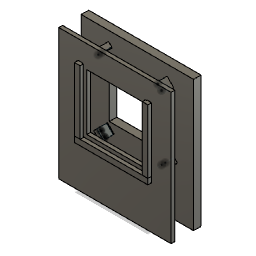
Target holder complete v23 (Autodesk Fusion 360 design; units mm, degrees)
Autodesk Fusion 360 part; units mm, degrees
sketch "Sketch1" plane through (0, 0, 0) normal (0, 0, 1) x (1, 0, 0) in component "Faceplate"
  line L0 (10, 10) -> (310, 10)
  line L1 (310, 10) -> (310, 360)
  line L2 (310, 360) -> (10, 360)
  line L3 (10, 360) -> (10, 10)
  line L4 (85, 300) -> (235, 300)
  line L5 (235, 300) -> (235, 150)
  line L6 (235, 150) -> (85, 150)
  line L7 (85, 150) -> (85, 300)
  dimension "d7" = 10
  dimension "d8" = 10
  dimension "d10" = 350
  dimension "d11" = 75
  dimension "d12" = 140
  dimension "d13" = 150
  dimension "d14" = 150
  dimension "d15" = 75
  constraint horizontal L0
  constraint vertical L1
  constraint horizontal L2
  constraint vertical L3
  constraint horizontal L4
  constraint vertical L5
  constraint horizontal L6
  constraint vertical L7
  measures "d7" horizontal distance of origin L0.start
  measures "d8" vertical distance of origin L0.start
  measures "d10" distance of L0.end L1.end
  measures "d11" horizontal distance of L0.start L6.end
  measures "d12" vertical distance of L0.start L6.end
  measures "d13" distance of L5.end L6.end
  measures "d14" distance of L4.end L5.end
  measures "d15" horizontal distance of L0.end L5.end
extrude "Extrude1" add sketch "Sketch1" against normal blind 10 makes body 1 in component "Faceplate"
sketch "Sketch2" plane through (0, 0, 0) normal (0, 0, 1) x (1, 0, 0) in component "Bottom holder"
  line L0 (235, 150) -> (85, 150)
  line L1 (85, 150) -> (85, 300)
  line L2 (85, 300) -> (235, 300)
  line L3 (235, 300) -> (235, 150)
  line L4 (10, 360) -> (10, 10)
  line L5 (10, 10) -> (310, 10)
  line L6 (310, 10) -> (310, 360)
  line L7 (310, 360) -> (10, 360)
  line L8 (258, 125) -> (62, 125)
  line L9 (62, 125) -> (62, 140)
  line L10 (62, 140) -> (258, 140)
  line L11 (258, 125) -> (258, 140)
  dimension "d18" = 196
  dimension "d20" = 15
  dimension "d69" = 10
  dimension "d70" = 23
  dimension "d74" = 15
  constraint horizontal L8
  constraint vertical L9
  constraint perpendicular L9 L10
  constraint perpendicular L10 L11
  measures "d18" distance of L8.start L8.end
  measures "d20" distance of L9.end L8.end
  measures "d69" vertical distance of L0.start L10.end
  measures "d70" horizontal distance of L0.end L9.end
  measures "d74" distance of L8.start L10.end
sketch "Sketch1 (2)" plane through (0, 0, 0) normal (0, 0, 1) x (1, 0, 0) in component "Left holder"
  line L0 (235, 150) -> (85, 150)
  line L1 (85, 150) -> (85, 300)
  line L2 (85, 300) -> (235, 300)
  line L3 (235, 300) -> (235, 150)
  line L4 (10, 360) -> (10, 10)
  line L5 (10, 10) -> (310, 10)
  line L6 (310, 10) -> (310, 360)
  line L7 (310, 360) -> (10, 360)
  line L8 (77, 310) -> (62, 310)
  line L9 (62, 310) -> (62, 140)
  line L10 (62, 140) -> (77, 140)
  line L11 (77, 140) -> (77, 310)
  dimension "d23" = 15
  dimension "d24" = 170
  dimension "d64" = 10
  dimension "d72" = 8
  constraint horizontal L8
  constraint vertical L9
  constraint horizontal L10
  constraint vertical L11
  measures "d23" distance of L8.start L8.end
  measures "d24" distance of L8.end L9.end
  measures "d64" vertical distance of L0.end L10.end
  measures "d72" horizontal distance of L1.end L8.start
sketch "Sketch1 (3)" plane through (0, 0, 0) normal (0, 0, 1) x (1, 0, 0) in component "Right holder"
  line L0 (235, 150) -> (85, 150)
  line L1 (85, 150) -> (85, 300)
  line L2 (85, 300) -> (241.0837, 300)
  line L3 (235, 300) -> (235, 150)
  line L4 (10, 360) -> (10, 10)
  line L5 (10, 10) -> (310, 10)
  line L6 (310, 10) -> (310, 360)
  line L7 (310, 360) -> (10, 360)
  line L8 (258, 310) -> (258, 140)
  line L9 (243, 140) -> (243, 310)
  line L10 (243, 140) -> (258, 140)
  line L11 (258, 310) -> (243, 310)
  dimension "d21" = 15
  dimension "d66" = 10
  dimension "d67" = 170
  dimension "d73" = 8
  constraint vertical L8
  constraint vertical L9
  constraint perpendicular L8 L10
  constraint perpendicular L9 L11
  measures "d21" distance of L9.end L8.start
  measures "d66" vertical distance of L0.start L9.start
  measures "d67" distance of L8.start L8.end
  measures "d73" horizontal distance of L3.start L9.end
extrude "Extrude2" add sketch "Sketch2" along normal blind 10 separate body contours L8 L9 L10 L11 makes body 2 in component "Bottom holder"
extrude "Extrude1'" add sketch "Sketch1 (2)" along normal blind 10 separate body contours L8 L9 L10 L11 makes body 3 in component "Left holder"
extrude "Extrude1''" add sketch "Sketch1 (3)" along normal blind 10 separate body contours L8 L9 L10 L11 makes body 4 in component "Right holder"
sketch "Sketch2 (2)" plane through (77, 0, 0) normal (1, 0, 0) x (0, 0, -1) in component "Left holder"
  line L0 (0, 140) -> (0, 310)
  line L1 (0, 310) -> (-10, 310)
  line L2 (-10, 310) -> (-10, 140)
  line L3 (-10, 140) -> (0, 140)
  line L4 (0, 310) -> (-1.5, 310)
  line L5 (-1.5, 310) -> (-1.5, 140)
  line L6 (-1.5, 140) -> (0, 140)
  line L7 (0, 140) -> (0, 310)
  dimension "d31" = 1.5
  constraint horizontal L4
  constraint vertical L5
  constraint horizontal L6
  constraint vertical L7
  constraint coincident L3 L5.end
  constraint coincident L0.end L1.start
  measures "d31" distance of L0.end L4.end
extrude "Extrude2'" cut sketch "Sketch2 (2)" against normal blind 3 contours L0 L1 L3 L4 L5 L6 L7 bodies 3 in component "Left holder"
sketch "Sketch2 (3)" plane through (243, 0, 0) normal (-1, 0, 0) x (0, 0, 1) in component "Right holder"
  line L0 (0, 310) -> (0, 140)
  line L1 (10, 140) -> (10, 310)
  line L2 (0, 310) -> (1.5, 310)
  line L3 (1.5, 310) -> (1.5, 145)
  line L4 (1.5, 145) -> (0, 145)
  line L5 (0, 145) -> (0, 310)
  line L6 (0, 140) -> (10, 140)
  line L7 (10, 310) -> (0, 310)
  dimension "d34" = 1.5
  constraint horizontal L2
  constraint vertical L3
  constraint horizontal L4
  constraint vertical L5
  constraint coincident L0.start L2.start
  measures "d34" distance of L3.end L4.end
extrude "Extrude2''" cut sketch "Sketch2 (3)" against normal blind 3 contours L0 L2 L3 L4 L5 L7 bodies 4 in component "Right holder"
sketch "Sketch3" plane through (0, 0, 0) normal (0, 0, -1) x (-1, 0, 0) in component "Bottom holder"
  line L0 (-258, 125) -> (-62, 125)
  line L1 (-62, 125) -> (-62, 140)
  circle A0 centre (-218, 132.5) radius 2.25
  circle A1 centre (-102, 132.5) radius 2.25
  line L2 (-62, 140) -> (-258, 140)
  line L3 (-258, 140) -> (-258, 125)
  dimension "d37" = 40
  dimension "d38" = 7.5
  dimension "d39" = 40
  dimension "d40" = 7.5
  dimension "d41" = 4.5
  dimension "d42" = 4.5
  measures "d37" horizontal distance of L0.start A0.centre
  measures "d38" vertical distance of L0.start A0.centre
  measures "d39" horizontal distance of L0.end A1.centre
  measures "d40" vertical distance of L0.end A1.centre
  measures "d41" diameter of A1
  measures "d42" diameter of A0
extrude "Extrude3" cut sketch "Sketch3" against normal blind 7 contours A0 | A1 bodies 2 in component "Bottom holder"
sketch "Sketch3 (2)" plane through (0, 0, 0) normal (0, 0, -1) x (-1, 0, 0) in component "Left holder"
  line L0 (-74, 310) -> (-74, 140)
  line L1 (-74, 140) -> (-62, 140)
  line L2 (-62, 140) -> (-62, 310)
  line L3 (-62, 310) -> (-74, 310)
  circle A0 centre (-68.5, 290) radius 2.25
  circle A1 centre (-68.5, 160) radius 2.25
  dimension "d45" = 20
  dimension "d46" = 20
  dimension "d47" = 6.5
  dimension "d48" = 6.5
  dimension "d49" = 4.5
  dimension "d50" = 4.5
  measures "d45" vertical distance of L2.end A0.centre
  measures "d46" vertical distance of L1.end A1.centre
  measures "d47" horizontal distance of L2.end A0.centre
  measures "d48" horizontal distance of L1.end A1.centre
  measures "d49" diameter of A0
  measures "d50" diameter of A1
sketch "Sketch3 (3)" plane through (0, 0, 0) normal (0, 0, -1) x (-1, 0, 0) in component "Right holder"
  line L0 (-246, 145) -> (-246, 310)
  line L1 (-258, 310) -> (-258, 140)
  circle A0 centre (-251.5, 290) radius 2.25
  circle A1 centre (-251.5, 160) radius 2.25
  line L2 (-246, 310) -> (-258, 310)
  line L3 (-258, 140) -> (-243, 140)
  line L4 (-243, 140) -> (-243, 145)
  line L5 (-243, 145) -> (-246, 145)
  dimension "d52" = 20
  dimension "d53" = 20
  dimension "d55" = 6.5
  dimension "d56" = 6.5
  dimension "d57" = 4.5
  dimension "d58" = 4.5
  measures "d52" vertical distance of L1.start A0.centre
  measures "d53" vertical distance of L1.end A1.centre
  measures "d55" horizontal distance of L1.start A0.centre
  measures "d56" horizontal distance of L1.end A1.centre
  measures "d57" diameter of A1
  measures "d58" diameter of A0
extrude "Extrude3'" cut sketch "Sketch3 (2)" against normal blind 7 contours A0 | A1 bodies 3 in component "Left holder"
extrude "Extrude3''" cut sketch "Sketch3 (3)" against normal blind 7 contours A0 | A1 bodies 4 in component "Right holder"
ref_plane "WorkPlane1" through (160, 185, -60) normal (0, 0, -1) x (-1, 0, 0) in component "Bottom holder"
sketch "Sketch1 (4)" plane through (160, 185, -60) normal (0, 0, -1) x (1, 0, 0) in component "Backplate"
  line L0 (150, -175) -> (-150, -175)
  line L1 (-150, -175) -> (-150, 175)
  line L2 (-150, 175) -> (150, 175)
  line L3 (150, 175) -> (150, -175)
  line L4 (75, -115) -> (-75, -115)
  line L5 (-75, -115) -> (-75, 35)
  line L6 (-75, 35) -> (75, 35)
  line L7 (75, 35) -> (75, -115)
  dimension "d76" = 300
  dimension "d77" = 350
  dimension "d78" = 175
  dimension "d79" = 150
  dimension "d84" = 150
  dimension "d85" = 150
  dimension "d86" = 75
  dimension "d87" = 60
  constraint horizontal L0
  constraint vertical L1
  constraint horizontal L2
  constraint vertical L3
  constraint horizontal L4
  constraint vertical L5
  constraint horizontal L6
  constraint vertical L7
  measures "d76" distance of L1.end L2.end
  measures "d77" distance of L0.start L2.end
  measures "d78" vertical distance of origin L1.end
  measures "d79" horizontal distance of origin L1.end
  measures "d84" distance of L4.start L6.end
  measures "d85" distance of L4.start L4.end
  measures "d86" distance of L3 L6.end
  measures "d87" distance of L0 L4.start
extrude "Extrude1'''" add sketch "Sketch1 (4)" along normal blind 20 separate body makes body 5 in component "Backplate"
sketch "Sketch1 (5)" plane through (0, 0, -60) normal (0, 0, 1) x (1, 0, 0) in component "Help lines"
  line L0 (235, 150) -> (85, 150)
  line L1 (85, 150) -> (85, 300)
  line L2 (85, 300) -> (235, 300)
  line L3 (235, 300) -> (235, 150)
  line L4 (10, 10) -> (310, 10)
  line L5 (310, 10) -> (310, 360)
  line L6 (310, 360) -> (10, 360)
  line L7 (10, 360) -> (10, 10)
  line L8 (85, 300) -> (235, 150)
  line L9 (85, 150) -> (235, 300)
  circle A0 centre (160, 225) radius 115
  dimension "d90" = 230
  constraint coincident L1.end L2.start
  constraint coincident L0.start L3.end
  constraint coincident L0.end L1.start
  constraint coincident L2.end L3.start
  constraint midpoint L8 A0.centre
  measures "d90" diameter of A0
sketch "Sketch2 (4)" plane through (0, 0, -60) normal (0, 0, 1) x (1, 0, 0) in component "Sensor-Holder West"
  line L0 (235, 150) -> (85, 150)
  line L1 (85, 150) -> (85, 300)
  line L2 (85, 300) -> (235, 300)
  line L3 (235, 300) -> (235, 150)
  line L4 (10, 10) -> (310, 10)
  line L5 (310, 10) -> (310, 360)
  line L6 (310, 360) -> (10, 360)
  line L7 (10, 360) -> (10, 10)
  line L8 (78.8806, 143.4853) -> (96.5583, 125.8076)
  line L9 (96.5583, 125.8076) -> (88.073, 117.3223)
  line L10 (88.073, 117.3223) -> (70.3954, 135)
  line L11 (70.3954, 135) -> (78.8806, 143.4853)
  circle A0 centre (160, 225) radius 115
  point P0 (85, 150)
  dimension "d91" = 12
  dimension "d92" = 25
  dimension "d93" = 15
  dimension "d94" = 45
  constraint perpendicular L8 L9
  constraint parallel L8 L10
  constraint parallel L9 L11
  constraint coincident L8.start A0
  measures "d91" distance of L8.start L10.end
  measures "d92" distance of L9.end L10.end
  measures "d93" vertical distance of L10.end P0
  measures "d94" angle of L7 L10
extrude "Extrude1''''" add sketch "Sketch2 (4)" along normal blind 27 separate body contours L8 L9 L10 L11 makes body 6 in component "Sensor-Holder West"
sketch "Sketch3 (4)" plane through (111.183, 111.183, 0) normal (0.707107, 0.707107, 0) x (0, 0, -1) in component "Sensor-Holder West"
  line L0 (60, 20.6824) -> (60, 45.6824)
  line L1 (60, 45.6824) -> (33, 45.6824)
  line L2 (33, 45.6824) -> (33, 20.6824)
  line L3 (33, 20.6824) -> (60, 20.6824)
  line L4 (60, 45.6824) -> (59, 45.6824)
  line L5 (59, 45.6824) -> (59, 20.6824)
  line L6 (59, 20.6824) -> (60, 20.6824)
  line L7 (60, 20.6824) -> (60, 45.6824)
  point P0 (60, 45.9619)
  dimension "d97" = 1
  constraint horizontal L4
  constraint vertical L5
  constraint horizontal L6
  constraint vertical L7
  constraint coincident L3 L5.end
  constraint coincident L0.end L1.start
  measures "d97" horizontal distance of L4.end P0
extrude "Extrude2'''" add sketch "Sketch3 (4)" along normal blind 2 contours L0 L1 L3 L4 L5 L6 L7 bodies 6 in component "Sensor-Holder West"
sketch "Sketch4" plane through (111.183, 111.183, 0) normal (0.707107, 0.707107, 0) x (0, 0, -1) in component "Sensor-Holder West"
  line L0 (59, 20.6824) -> (59, 45.6824)
  line L1 (59, 45.6824) -> (33, 45.6824)
  line L2 (33, 45.6824) -> (33, 20.6824)
  line L3 (33, 20.6824) -> (59, 20.6824)
  circle A0 centre (38.5, 38.6824) radius 1.5
  circle A1 centre (38.5, 24.6824) radius 1.5
  dimension "d100" = 3
  dimension "d101" = 3
  dimension "d102" = 14
  dimension "d103" = 20.5
  dimension "d104" = 7
  dimension "d105" = 20.5
  measures "d100" diameter of A0
  measures "d101" diameter of A1
  measures "d102" distance of A0.centre A1.centre
  measures "d103" horizontal distance of L0.end A0.centre
  measures "d104" vertical distance of L1.end A0.centre
  measures "d105" horizontal distance of L0.start A1.centre
extrude "Extrude3'''" add sketch "Sketch4" along normal blind 3 contours A0 bodies 6 in component "Sensor-Holder West"
extrude "Extrude4" add sketch "Sketch4" along normal up to surface (3 mm away) contours A1 bodies 6 in component "Sensor-Holder West"
sketch "Sketch2 (5)" plane through (0, 0, -60) normal (0, 0, 1) x (1, 0, 0) in component "Sensor-Holder East"
  line L0 (235, 150) -> (85, 150)
  line L1 (85, 150) -> (85, 300)
  line L2 (85, 300) -> (235, 300)
  line L3 (235, 300) -> (235, 150)
  line L4 (10, 10) -> (310, 10)
  line L5 (310, 10) -> (310, 360)
  line L6 (310, 360) -> (10, 360)
  line L7 (10, 360) -> (10, 10)
  line L8 (78.8806, 143.4853) -> (96.5583, 125.8076)
  line L9 (96.5583, 125.8076) -> (88.073, 117.3223)
  line L10 (88.073, 117.3223) -> (70.3954, 135)
  line L11 (70.3954, 135) -> (78.8806, 143.4853)
  circle A0 centre (160, 225) radius 115
  point P0 (85, 150)
  dimension "d91_1" = 12
  dimension "d92_1" = 25
  dimension "d93_1" = 15
  dimension "d94_1" = 45
  constraint perpendicular L8 L9
  constraint parallel L8 L10
  constraint parallel L9 L11
  constraint coincident L8.start A0
  measures "d91_1" distance of L8.start L10.end
  measures "d92_1" distance of L9.end L10.end
  measures "d93_1" vertical distance of L10.end P0
  measures "d94_1" angle of L7 L10
extrude "Extrude1'''''" add sketch "Sketch2 (5)" along normal blind 27 separate body contours L8 L9 L10 L11 makes body 7 in component "Sensor-Holder East"
sketch "Sketch3 (5)" plane through (111.183, 111.183, 0) normal (0.707107, 0.707107, 0) x (0, 0, -1) in component "Sensor-Holder East"
  line L0 (60, 20.6824) -> (60, 45.6824)
  line L1 (60, 45.6824) -> (33, 45.6824)
  line L2 (33, 45.6824) -> (33, 20.6824)
  line L3 (33, 20.6824) -> (60, 20.6824)
  line L4 (60, 45.6824) -> (59, 45.6824)
  line L5 (59, 45.6824) -> (59, 20.6824)
  line L6 (59, 20.6824) -> (60, 20.6824)
  line L7 (60, 20.6824) -> (60, 45.6824)
  point P0 (60, 45.9619)
  dimension "d97_1" = 1
  constraint horizontal L4
  constraint vertical L5
  constraint horizontal L6
  constraint vertical L7
  constraint coincident L3 L5.end
  constraint coincident L0.end L1.start
  measures "d97_1" horizontal distance of L4.end P0
extrude "Extrude2''''" add sketch "Sketch3 (5)" along normal blind 2 contours L0 L1 L3 L4 L5 L6 L7 bodies 7 in component "Sensor-Holder East"
sketch "Sketch4 (2)" plane through (111.183, 111.183, 0) normal (0.707107, 0.707107, 0) x (0, 0, -1) in component "Sensor-Holder East"
  line L0 (59, 20.6824) -> (59, 45.6824)
  line L1 (59, 45.6824) -> (33, 45.6824)
  line L2 (33, 45.6824) -> (33, 20.6824)
  line L3 (33, 20.6824) -> (59, 20.6824)
  circle A0 centre (38.5, 38.6824) radius 1.5
  circle A1 centre (38.5, 24.6824) radius 1.5
  dimension "d100_1" = 3
  dimension "d101_1" = 3
  dimension "d102_1" = 14
  dimension "d103_1" = 20.5
  dimension "d104_1" = 7
  dimension "d105_1" = 20.5
  measures "d100_1" diameter of A0
  measures "d101_1" diameter of A1
  measures "d102_1" distance of A0.centre A1.centre
  measures "d103_1" horizontal distance of L0.end A0.centre
  measures "d104_1" vertical distance of L1.end A0.centre
  measures "d105_1" horizontal distance of L0.start A1.centre
extrude "Extrude3''''" add sketch "Sketch4 (2)" along normal blind 3 contours A0 bodies 7 in component "Sensor-Holder East"
extrude "Extrude4'" add sketch "Sketch4 (2)" along normal up to surface (3 mm away) contours A1 bodies 7 in component "Sensor-Holder East"
move_body "Move1" bodies 7 to x (1, 0, 0) y (0, 1, 0) z (0, 0, 1) at (2.1213, 2.1213, 0) in component "Sensor-Holder East"
sketch "Sketch2 (6)" plane through (0, 0, -60) normal (0, 0, 1) x (1, 0, 0) in component "Sensor-Holder South"
  line L0 (235, 150) -> (85, 150)
  line L1 (85, 150) -> (85, 300)
  line L2 (85, 300) -> (235, 300)
  line L3 (235, 300) -> (235, 150)
  line L4 (10, 10) -> (310, 10)
  line L5 (310, 10) -> (310, 360)
  line L6 (310, 360) -> (10, 360)
  line L7 (10, 360) -> (10, 10)
  line L8 (78.8806, 143.4853) -> (96.5583, 125.8076)
  line L9 (96.5583, 125.8076) -> (88.073, 117.3223)
  line L10 (88.073, 117.3223) -> (70.3954, 135)
  line L11 (70.3954, 135) -> (78.8806, 143.4853)
  circle A0 centre (160, 225) radius 115
  point P0 (85, 150)
  dimension "d91_2" = 12
  dimension "d92_2" = 25
  dimension "d93_2" = 15
  dimension "d94_2" = 45
  constraint perpendicular L8 L9
  constraint parallel L8 L10
  constraint parallel L9 L11
  constraint coincident L8.start A0
  measures "d91_2" distance of L8.start L10.end
  measures "d92_2" distance of L9.end L10.end
  measures "d93_2" vertical distance of L10.end P0
  measures "d94_2" angle of L7 L10
extrude "Extrude1''''''" add sketch "Sketch2 (6)" along normal blind 27 separate body contours L8 L9 L10 L11 makes body 8 in component "Sensor-Holder South"
sketch "Sketch3 (6)" plane through (111.183, 111.183, 0) normal (0.707107, 0.707107, 0) x (0, 0, -1) in component "Sensor-Holder South"
  line L0 (60, 20.6824) -> (60, 45.6824)
  line L1 (60, 45.6824) -> (33, 45.6824)
  line L2 (33, 45.6824) -> (33, 20.6824)
  line L3 (33, 20.6824) -> (60, 20.6824)
  line L4 (60, 45.6824) -> (59, 45.6824)
  line L5 (59, 45.6824) -> (59, 20.6824)
  line L6 (59, 20.6824) -> (60, 20.6824)
  line L7 (60, 20.6824) -> (60, 45.6824)
  point P0 (60, 45.9619)
  dimension "d97_2" = 1
  constraint horizontal L4
  constraint vertical L5
  constraint horizontal L6
  constraint vertical L7
  constraint coincident L3 L5.end
  constraint coincident L0.end L1.start
  measures "d97_2" horizontal distance of L4.end P0
extrude "Extrude2'''''" add sketch "Sketch3 (6)" along normal blind 2 contours L0 L1 L3 L4 L5 L6 L7 bodies 8 in component "Sensor-Holder South"
sketch "Sketch4 (3)" plane through (111.183, 111.183, 0) normal (0.707107, 0.707107, 0) x (0, 0, -1) in component "Sensor-Holder South"
  line L0 (59, 20.6824) -> (59, 45.6824)
  line L1 (59, 45.6824) -> (33, 45.6824)
  line L2 (33, 45.6824) -> (33, 20.6824)
  line L3 (33, 20.6824) -> (59, 20.6824)
  circle A0 centre (38.5, 38.6824) radius 1.5
  circle A1 centre (38.5, 24.6824) radius 1.5
  dimension "d100_2" = 3
  dimension "d101_2" = 3
  dimension "d102_2" = 14
  dimension "d103_2" = 20.5
  dimension "d104_2" = 7
  dimension "d105_2" = 20.5
  measures "d100_2" diameter of A0
  measures "d101_2" diameter of A1
  measures "d102_2" distance of A0.centre A1.centre
  measures "d103_2" horizontal distance of L0.end A0.centre
  measures "d104_2" vertical distance of L1.end A0.centre
  measures "d105_2" horizontal distance of L0.start A1.centre
extrude "Extrude3'''''" add sketch "Sketch4 (3)" along normal blind 3 contours A0 bodies 8 in component "Sensor-Holder South"
extrude "Extrude4''" add sketch "Sketch4 (3)" along normal up to surface (3 mm away) contours A1 bodies 8 in component "Sensor-Holder South"
sketch "Sketch2 (7)" plane through (0, 0, -60) normal (0, 0, 1) x (1, 0, 0) in component "Sensor-Holder North"
  line L0 (235, 150) -> (85, 150)
  line L1 (85, 150) -> (85, 300)
  line L2 (85, 300) -> (235, 300)
  line L3 (235, 300) -> (235, 150)
  line L4 (10, 10) -> (310, 10)
  line L5 (310, 10) -> (310, 360)
  line L6 (310, 360) -> (10, 360)
  line L7 (10, 360) -> (10, 10)
  line L8 (78.8806, 143.4853) -> (96.5583, 125.8076)
  line L9 (96.5583, 125.8076) -> (88.073, 117.3223)
  line L10 (88.073, 117.3223) -> (70.3954, 135)
  line L11 (70.3954, 135) -> (78.8806, 143.4853)
  circle A0 centre (160, 225) radius 115
  point P0 (85, 150)
  dimension "d91_3" = 12
  dimension "d92_3" = 25
  dimension "d93_3" = 15
  dimension "d94_3" = 45
  constraint perpendicular L8 L9
  constraint parallel L8 L10
  constraint parallel L9 L11
  constraint coincident L8.start A0
  measures "d91_3" distance of L8.start L10.end
  measures "d92_3" distance of L9.end L10.end
  measures "d93_3" vertical distance of L10.end P0
  measures "d94_3" angle of L7 L10
extrude "Extrude1'''''''" add sketch "Sketch2 (7)" along normal blind 27 separate body contours L8 L9 L10 L11 makes body 9 in component "Sensor-Holder North"
sketch "Sketch3 (7)" plane through (111.183, 111.183, 0) normal (0.707107, 0.707107, 0) x (0, 0, -1) in component "Sensor-Holder North"
  line L0 (60, 20.6824) -> (60, 45.6824)
  line L1 (60, 45.6824) -> (33, 45.6824)
  line L2 (33, 45.6824) -> (33, 20.6824)
  line L3 (33, 20.6824) -> (60, 20.6824)
  line L4 (60, 45.6824) -> (59, 45.6824)
  line L5 (59, 45.6824) -> (59, 20.6824)
  line L6 (59, 20.6824) -> (60, 20.6824)
  line L7 (60, 20.6824) -> (60, 45.6824)
  point P0 (60, 45.9619)
  dimension "d97_3" = 1
  constraint horizontal L4
  constraint vertical L5
  constraint horizontal L6
  constraint vertical L7
  constraint coincident L3 L5.end
  constraint coincident L0.end L1.start
  measures "d97_3" horizontal distance of L4.end P0
extrude "Extrude2''''''" add sketch "Sketch3 (7)" along normal blind 2 contours L0 L1 L3 L4 L5 L6 L7 bodies 9 in component "Sensor-Holder North"
sketch "Sketch4 (4)" plane through (111.183, 111.183, 0) normal (0.707107, 0.707107, 0) x (0, 0, -1) in component "Sensor-Holder North"
  line L0 (59, 20.6824) -> (59, 45.6824)
  line L1 (59, 45.6824) -> (33, 45.6824)
  line L2 (33, 45.6824) -> (33, 20.6824)
  line L3 (33, 20.6824) -> (59, 20.6824)
  circle A0 centre (38.5, 38.6824) radius 1.5
  circle A1 centre (38.5, 24.6824) radius 1.5
  dimension "d100_3" = 3
  dimension "d101_3" = 3
  dimension "d102_3" = 14
  dimension "d103_3" = 20.5
  dimension "d104_3" = 7
  dimension "d105_3" = 20.5
  measures "d100_3" diameter of A0
  measures "d101_3" diameter of A1
  measures "d102_3" distance of A0.centre A1.centre
  measures "d103_3" horizontal distance of L0.end A0.centre
  measures "d104_3" vertical distance of L1.end A0.centre
  measures "d105_3" horizontal distance of L0.start A1.centre
extrude "Extrude3''''''" add sketch "Sketch4 (4)" along normal blind 3 contours A0 bodies 9 in component "Sensor-Holder North"
extrude "Extrude4'''" add sketch "Sketch4 (4)" along normal up to surface (3 mm away) contours A1 bodies 9 in component "Sensor-Holder North"
component "Bottom holder" placed x (1, 0, 0) y (0, 1, 0) z (0, 0, 1) at (0, 0, 0)
component "Left holder" placed x (1, 0, 0) y (0, 1, 0) z (0, 0, 1) at (0, 0, 0)
component "Right holder" placed x (1, 0, 0) y (0, 1, 0) z (0, 0, 1) at (0, 0, 0)
component "Faceplate" placed x (1, 0, 0) y (0, 1, 0) z (0, 0, 1) at (0, 0, 0)
component "Backplate" placed x (1, 0, 0) y (0, 1, 0) z (0, 0, 1) at (0, 0, 0)
component "Sensor-Holder West" placed x (1, 0, 0) y (0, 1, 0) z (0, 0, 1) at (0, 0, 0)
component "Help lines" placed x (1, 0, 0) y (0, 1, 0) z (0, 0, 1) at (0, 0, 0)
component "Sensor-Holder East" placed x (1, 0, 0) y (0, 1, 0) z (0, 0, 1) at (0, 0, 0)
component "Sensor-Holder South" placed x (1, 0, 0) y (0, 1, 0) z (0, 0, 1) at (0, 0, 0)
component "Sensor-Holder North" placed x (1, 0, 0) y (0, 1, 0) z (0, 0, 1) at (0, 0, 0)
